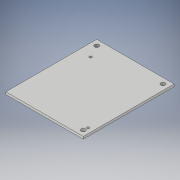
# Autodesk Inventor part: top
Saved by Autodesk Inventor 2018.1 (Build 221171000, 171)
## iProperties
Created: 2022-03-02
Part Number: top
Material: Generic
Document SubType Name: Modeling
Designer: micha
Density: 1 g/cm^3
Appearance: Default
Author: micha
Autodesk Inventor part; units mm, degrees
ref_plane "YZ Plane" through (0, 0, 0) normal (1, 0, 0) x (0, 1, 0)
ref_plane "XZ Plane" through (0, 0, 0) normal (0, 1, 0) x (-1, 0, 0)
ref_plane "XY Plane" through (0, 0, 0) normal (0, 0, 1) x (1, 0, 0)
sketch "Sketch1" plane through (0, 0, 0) normal (0, 1, 0) x (-1, 0, 0)
  line L0 (0, 0) -> (-63, 0)
  line L1 (-63, 0) -> (-63, -74)
  line L2 (-63, -74) -> (0, -74)
  line L3 (0, -74) -> (0, 0)
  dimension "d0" = 63
  dimension "d1" = 74
  constraints: 8 end point, 2 parallel, 1 horizontal, 1 perpendicular
  measures "d0" distance of L2.end L1.end
  measures "d1" distance of L1.end L0.end
extrude "Extrusion1" add sketch "Sketch1" along normal blind 2
sketch "Sketch2" plane through (0, 2, 0) normal (0, 1, 0) x (1, 0, 0)
  circle A0 centre (59, 8) radius 1
  line L0 (0, 0) -> (63, 0) projected
  line L1 (63, 0) -> (63, 74) projected
  circle A1 centre (10, 59) radius 1
  line L2 (63, 74) -> (0, 74) projected
  line L3 (0, 74) -> (0, 0) projected
  dimension "d4" = 2
  dimension "d5" = 8
  dimension "d6" = 4
  dimension "d7" = 2
  dimension "d8" = 15
  dimension "d9" = 10
  constraints: 2 centre point
  measures "d4" diameter of A0
  measures "d5" distance from line of L0 A0.centre
  measures "d6" distance from line of L1 A0.centre
  measures "d7" diameter of A1
  measures "d8" distance from line of L2 A1.centre
  measures "d9" distance from line of L3 A1.centre
extrude "Extrusion2" cut sketch "Sketch2" against normal up to next contours A0 | A1
sketch "Sketch3" plane through (0, 0, 0) normal (0, -1, 0) x (1, 0, 0)
  line L0 (2.25, -2.25) -> (60.75, -2.25)
  line L1 (60.75, -2.25) -> (60.75, -71.75)
  line L2 (60.75, -71.75) -> (2.25, -71.75)
  line L3 (2.25, -71.75) -> (2.25, -2.25)
  line L4 (0, 0) -> (63, 0) projected
  line L5 (0, -74) -> (0, 0) projected
  line L6 (3.25, -3.25) -> (59.75, -3.25)
  line L7 (59.75, -3.25) -> (59.75, -70.75)
  line L8 (59.75, -70.75) -> (3.25, -70.75)
  line L9 (3.25, -70.75) -> (3.25, -3.25)
  dimension "d12" = 58.5
  dimension "d13" = 69.5
  dimension "d14" = 2.25
  dimension "d15" = 2.25
  dimension "d16" = 56.5
  dimension "d17" = 67.5
  dimension "d18" = 1
  dimension "d19" = 1
  constraints: 16 end point, 4 parallel, 2 horizontal, 2 perpendicular
  measures "d12" distance of L1.end L2.end
  measures "d13" distance of L0.end L1.end
  measures "d14" distance between parallel lines of L4 L0
  measures "d15" distance between parallel lines of L5 L3
  measures "d16" distance of L7.end L8.end
  measures "d17" distance of L6.end L7.end
  measures "d18" distance between parallel lines of L0 L6
  measures "d19" distance between parallel lines of L3 L9
extrude "Extrusion3" add sketch "Sketch3" along normal blind 1
chamfer "Chamfer1" distance 1 angle 45 1 edges at (3.25, -1, -37) measured on face at (3.25, -0.3333, -48.25)
chamfer "Chamfer2" distance 1 angle 45 1 edges at (31.5, -1, -3.25) measured on face at (40.9167, -0.3335, -3.25)
chamfer "Chamfer3" distance 1 angle 45 1 edges at (59.75, -1, -37) measured on face at (59.75, -0.6667, -27.5538)
chamfer "Chamfer4" distance 1 angle 45 1 edges at (31.5, -1, -70.75) measured on face at (22.0833, -0.6668, -70.75)
sketch "Sketch4" plane through (0, 2, 0) normal (0, 1, 0) x (1, 0, 0)
  circle A0 centre (4.5, 69.5) radius 1.75
  line L0 (63, 74) -> (0, 74) projected
  line L1 (0, 74) -> (0, 0) projected
  circle A1 centre (58.5, 69.5) radius 1.75
  line L2 (63, 0) -> (63, 74) projected
  circle A2 centre (58.5, 4.5) radius 1.75
  line L3 (0, 0) -> (63, 0) projected
  dimension "d34" = 3.5
  dimension "d35" = 4.5
  dimension "d36" = 4.5
  dimension "d37" = 3.5
  dimension "d38" = 4.5
  dimension "d39" = 4.5
  dimension "d40" = 3.5
  dimension "d41" = 4.5
  dimension "d42" = 4.5
  constraints: 3 centre point
  measures "d34" diameter of A0
  measures "d35" distance from line of L0 A0.centre
  measures "d36" distance from line of L1 A0.centre
  measures "d37" diameter of A1
  measures "d38" distance from line of L0 A1.centre
  measures "d39" distance from line of L2 A1.centre
  measures "d40" diameter of A2
  measures "d41" distance from line of L3 A2.centre
  measures "d42" distance from line of L2 A2.centre
extrude "Extrusion4" cut sketch "Sketch4" against normal up to next contours A0 | A1 | A2
body "Solid1"
